Autodesk Inventor part; units mm, degrees
(part 3 of 3)
  line L461 (85.6298, 87) -> (78.6298, 87) construction
  line L462 (78.6298, 87) -> (78.6298, 77) construction
  line L463 (78.6298, 77) -> (85.6298, 77) construction
  line L464 (85.6298, 92) -> (85.6298, 102) construction
  line L465 (85.6298, 102) -> (78.6298, 102) construction
  line L466 (78.6298, 102) -> (78.6298, 92) construction
  line L467 (78.6298, 92) -> (85.6298, 92) construction
  line L468 (85.6298, 107) -> (85.6298, 117) construction
  line L469 (85.6298, 117) -> (78.6298, 117) construction
  line L470 (78.6298, 117) -> (78.6298, 107) construction
  line L471 (78.6298, 107) -> (85.6298, 107) construction
  line L472 (75.6298, 230.325) -> (75.6298, 122) projected
  line L473 (75.6298, 122) -> (138.6298, 122) projected
  line L474 (138.6298, 122) -> (138.6298, 0) projected
  line L475 (104.6298, 2) -> (111.6298, 2) construction
  line L476 (111.6298, 2) -> (111.6298, 12) construction
  line L477 (111.6298, 12) -> (104.6298, 12) construction
  line L478 (104.6298, 12) -> (104.6298, 2) construction
  line L479 (-0.7738, 0) -> (138.6298, 0) projected
  line L480 (39.6298, 2) -> (46.6298, 2) construction
  line L481 (46.6298, 2) -> (46.6298, 12) construction
  line L482 (46.6298, 12) -> (39.6298, 12) construction
  line L483 (39.6298, 12) -> (39.6298, 2) construction
  line L484 (-0.7738, 146.3758) -> (-0.7738, 0) projected
  line L485 (36.7399, 0) -> (41.3233, 0)
  line L486 (109.9362, 0) -> (114.5196, 0)
  point P0 (75.6298, 165)
  dimension "d594" = 20
  dimension "d595" = 38
  constraints: 22 end point, 6 parallel, 5 point on line, 3 perpendicular, 2 horizontal, 1 coincident, 1 midpoint, 1 vertical alignment
  measures "d594" distance between parallel lines of L2 L0
  measures "d595" distance between parallel lines of L3 L1
sketch "Эскиз114" plane through (0, -165, -85) normal (0, -1, 0) x (1, 0, 0)
  line L0 (32, 66) -> (32, 22) construction
  line L1 (32, 22) -> (34, 22) projected
  line L2 (34, 66) -> (34, 22) construction
  line L3 (34, 66) -> (32, 66) construction
  line L4 (32, 22) -> (34, 22)
  line L5 (34, 22) -> (34, 23)
  line L6 (34, 23) -> (32, 23)
  line L7 (32, 23) -> (32, 22)
  point P0 (0, 85)
  dimension "d601" = 1
  constraints: 8 end point, 2 parallel, 1 horizontal, 1 perpendicular, 1 point on line
  measures "d601" distance between parallel lines of L6 L1
sketch "Эскиз115" plane through (34, -165, 76.4035) normal (1, 0, 0) x (0, 0, -1)
  line L0 (76.4035, 230.325) -> (76.4035, 228.825)
  arc A0 (76.4035, 228.825) -> (0, 146.3758) centre (85.719, 143.5674) ccw
  arc A1 (76.4035, 230.325) -> (0, 146.3758) centre (74.3088, 155.4888) ccw
  point P0 (76.4035, 165)
  dimension "d604" = 1.5
  constraints: 4 point on circle, 2 centre point, 2 end point, 1 coincident, 1 vertical
  measures "d604" distance of L0.start L0.end
sketch "Эскиз116" plane through (0, -165, -85) normal (0, -1, 0) x (1, 0, 0)
  line L0 (32, 104) -> (34, 104) projected
  line L1 (32, 104) -> (34, 104)
  line L2 (34, 104) -> (34, 105.5)
  line L3 (34, 105.5) -> (32, 105.5)
  line L4 (32, 105.5) -> (32, 104)
  point P0 (0, 85)
  dimension "d607" = 1.5
  dimension "d10" = 170
  dimension "d15" = 4
  dimension "d16" = 35
  dimension "d97" = 2
  constraints: 10 end point, 3 point on circle, 2 horizontal, 2 vertical alignment, 1 centre point, 1 horizontal alignment, 1 perpendicular, 1 vertical
  measures "d10" distance of L0.start L0.end
  measures "d16" distance from line of point (0, 0) L3
  measures "d97" distance of L4.start L4.end
